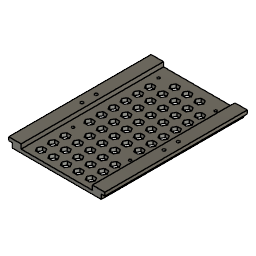
powersupply mount (Autodesk Fusion 360 design; units mm, degrees)
Autodesk Fusion 360 part; units mm, degrees
sketch "Szkic1" plane through (0, 0, 0) normal (0, 0, 1) x (1, 0, 0)
  line L0 (38.5639, 59) -> (-38.5639, 59)
  line L1 (-39, 58.5639) -> (-39, -58.5639)
  line L2 (-38.5639, -59) -> (38.5639, -59)
  line L3 (39, -58.5639) -> (39, 58.5639)
  line L4 (39, 59) -> (-39, -59) construction
  line L5 (-39, 59) -> (38.8118, -58.7152) construction
  line L6 (38.5639, 61) -> (-38.5639, 61)
  line L7 (-41, 58.5639) -> (-41, -58.5639)
  line L8 (-38.5639, -61) -> (38.5639, -61)
  line L9 (41, -58.5639) -> (41, 58.5639)
  line L10 (41, 61) -> (-41, -61) construction
  line L11 (-41, 61) -> (41, -61) construction
  line L12 (-41, 61) -> (-41, 77)
  line L13 (41, 61) -> (41, 77)
  line L14 (41, 77) -> (50, 77)
  line L15 (-41, 77) -> (-50, 77)
  line L16 (-50, 77) -> (50, 77)
  line L17 (50, 77) -> (50, -123)
  line L18 (50, -123) -> (-50, -123)
  line L19 (-50, -123) -> (-50, 77)
  circle A0 centre (-40, -60) radius 1.75
  circle A1 centre (40, -60) radius 1.75
  circle A2 centre (40, 60) radius 1.75
  circle A3 centre (-40, 60) radius 1.75
  line L20 (-67.5, -123) -> (-67.5, 77)
  line L21 (67.5, 77) -> (67.5, -123)
  line L22 (66.42, -123) -> (-67.5, 125) construction
  line L23 (-67.5, -125) -> (67.5, 125) construction
  line L24 (-67.5, 77) -> (67.5, 77)
  line L25 (-67.5, -123) -> (67.5, -123)
  line L26 (67.5, 77) -> (67.5, -123)
  line L27 (67.5, -123) -> (62.5, -123)
  line L28 (62.5, -123) -> (62.5, 77)
  line L29 (62.5, 77) -> (67.5, 77)
  line L30 (-67.5, -123) -> (-67.5, 77)
  line L31 (-67.5, 77) -> (-62.5, 77)
  line L32 (-62.5, 77) -> (-62.5, -123)
  line L33 (-62.5, -123) -> (-67.5, -123)
  dimension "d1" = 118
  dimension "d3" = 122
  dimension "d4" = 82
  dimension "d5" = 16
  dimension "d6" = 16
  dimension "d7" = 9
  dimension "d8" = 9
  dimension "d9" = 200
  dimension "d10" = 3.5
  dimension "d11" = 3.5
  dimension "d12" = 3.5
  dimension "d13" = 3.5
  dimension "d14" = 135
  dimension "d15" = 5
  dimension "d16" = 5
  constraint horizontal L0
  constraint perpendicular L0 L1
  constraint parallel L0 L2
  constraint parallel L1 L3
  constraint coincident L4 origin
  constraint coincident L5 origin
  constraint horizontal L6
  constraint perpendicular L6 L7
  constraint parallel L6 L8
  constraint parallel L7 L9
  constraint coincident L10 origin
  constraint coincident L11 origin
  constraint perpendicular L6 L12
  constraint perpendicular L6 L13
  constraint perpendicular L13 L14
  constraint perpendicular L12 L15
  constraint perpendicular L16 L17
  constraint parallel L16 L18
  constraint parallel L17 L19
  constraint coincident A0 L2.start
  constraint coincident A0 L1.end
  constraint coincident A0 L8.start
  constraint coincident A0 L7.end
  constraint coincident A1 L8.end
  constraint coincident A1 L9.start
  constraint coincident A1 L2.end
  constraint coincident A1 L5.end
  constraint coincident A1 L3.start
  constraint coincident A2 L3.end
  constraint coincident A2 L0.start
  constraint coincident A2 L6.start
  constraint coincident A2 L9.end
  constraint coincident A3 L1.start
  constraint coincident A3 L0.end
  constraint coincident A3 L7.start
  constraint coincident A3 L6.end
  constraint parallel L20 L21
  constraint coincident L22 origin
  constraint coincident L23 origin
  constraint perpendicular L21 L24
  constraint perpendicular L21 L25
  constraint coincident L25 L22.start
  constraint perpendicular L26 L27
  constraint parallel L26 L28
  constraint parallel L27 L29
  constraint perpendicular L30 L31
  constraint parallel L30 L32
  constraint parallel L31 L33
  measures "d1" distance of L5.start L4.end
  measures "d3" distance of L11.start L10.end
  measures "d4" distance of L10.end L11.end
  measures "d5" distance of L11.start L12.end
  measures "d6" distance of L10.start L13.end
  measures "d7" distance of L13.end L14.end
  measures "d8" distance of L12.end L15.end
  measures "d9" distance of L15.end L18.end
  measures "d10" diameter of A0
  measures "d11" diameter of A1
  measures "d12" diameter of A2
  measures "d13" diameter of A3
  measures "d14" distance of L22.end L23.end
  measures "d15" distance of L21.start L28.end
  measures "d16" distance of L20.start L32.end
extrude "Wyciągnięcie proste1" add sketch "Szkic1" along normal blind 4 contours L0 L1 L2 L3 A0 A1 A2 A3 | L0 L6 A2 A3 | L6 L12 L13 L16 A2 A3 L24 | L3 L9 A1 A2 | L1 L7 A0 A3 | L7 L8 L9 L12 L13 L14 L15 L16 L17 L18 L19 A0 A1 A2 A3 L24 L25 | L2 L8 A0 A1
extrude "Wyciągnięcie proste2" add 1 faces at (-13, 19.5213, 4) along direction (0, 0, 1) blind 2
extrude "Wyciągnięcie proste3" add sketch "Szkic1" along normal blind 12.5 contours L17 L24 L25 L28 | L19 L24 L25 L32 | L21 L24 L25 L26 L27 L28 L29 | L20 L24 L25 L30 L31 L32 L33
extrude "Wyciągnięcie proste4" cut sketch "Szkic1" along normal blind 7.5 contours L21 L24 L25 L26 L27 L28 L29 | L20 L24 L25 L30 L31 L32 L33
extrude "Wyciągnięcie proste5" cut 1 faces at (-13.0417, 19.4948, 0) along direction (0, 0, 1) blind 1
sketch "Szkic2" plane through (0, 0, 1) normal (0, 0, -1) x (1, 0, 0)
  line L0 (-62.5, 123) -> (-62.5, -77)
  line L1 (-62.5, -77) -> (62.5, -77)
  line L2 (62.5, -77) -> (62.5, 123)
  line L3 (62.5, 123) -> (-62.5, 123)
  circle A0 centre (-40, 60) radius 1.75
  circle A1 centre (40, -60) radius 1.75
  circle A2 centre (40, 60) radius 1.75
  circle A3 centre (-40, -60) radius 1.75
  circle A4 centre (-40, -60) radius 3
  circle A5 centre (40, -60) radius 3
  circle A6 centre (-40, 60) radius 3
  circle A7 centre (40, 60) radius 3
  dimension "d27" = 6
  dimension "d28" = 6
  dimension "d29" = 6
  dimension "d30" = 6
  constraint concentric A3 A4
  constraint concentric A1 A5
  constraint concentric A0 A6
  constraint concentric A2 A7
  measures "d27" diameter of A4
  measures "d28" diameter of A5
  measures "d29" diameter of A6
  measures "d30" diameter of A7
extrude "Wyciągnięcie proste6" cut sketch "Szkic2" against normal blind 2.4 contours A4 | A5 | A6 | A7
sketch "Szkic3" plane through (0, 0, 12.5) normal (0, 0, 1) x (-1, 0, 0)
  line L0 (50, 123) -> (50, -77)
  line L1 (50, -77) -> (67.5, -77)
  line L2 (67.5, -77) -> (67.5, 123)
  line L3 (67.5, 123) -> (50, 123)
  line L4 (50, 5) -> (60, 5)
  line L5 (50, 35) -> (50, 5)
  line L6 (60, 5) -> (62, 7)
  line L7 (62, 7) -> (62, 33)
  line L8 (62, 33) -> (60, 35)
  line L9 (60, 35) -> (50, 35)
  line L10 (-50, 35) -> (-60, 35)
  line L11 (-50, 5) -> (-50, 35)
  line L12 (-60, 35) -> (-62, 33)
  line L13 (-62, 33) -> (-62, 7)
  line L14 (-62, 7) -> (-60, 5)
  line L15 (-60, 5) -> (-50, 5)
  circle A0 centre (57.5, 30) radius 2
  circle A1 centre (57.5, 10) radius 2
  circle A2 centre (-57.5, 30) radius 2
  circle A3 centre (-57.5, 10) radius 2
  dimension "d33" = 4
  dimension "d34" = 4
  dimension "d35" = 4
  dimension "d36" = 4
  measures "d33" diameter of A0
  measures "d34" diameter of A1
  measures "d35" diameter of A2
  measures "d36" diameter of A3
extrude "Wyciągnięcie proste7" cut sketch "Szkic3" against normal blind 8 contours A0 | A1 | A2 | A3
extrude "Wyciągnięcie proste8" cut 2 faces at (58.3333, -92.6667, 12.5) (-58.3333, -92.6667, 12.5) along direction (0, 0, -1) blind 0.2
sketch "Szkic4" plane through (0, 0, 1) normal (0, 0, -1) x (1, 0, 0)
  circle A0 centre (-40, 60) radius 3
  circle A1 centre (-40, -60) radius 3
  circle A2 centre (40, 60) radius 3
  circle A3 centre (40, -60) radius 3
  line L0 (-62.5, 123) -> (-62.5, -77)
  line L1 (-62.5, -77) -> (62.5, -77)
  line L2 (62.5, -77) -> (62.5, 123)
  line L3 (62.5, 123) -> (-62.5, 123)
  line L4 (-2.8868, 30) -> (-5.7735, 25)
  line L5 (-5.7735, 25) -> (-2.8868, 20)
  line L6 (-2.8868, 20) -> (2.8868, 20)
  line L7 (2.8868, 20) -> (5.7735, 25)
  line L8 (5.7735, 25) -> (2.8868, 30)
  line L9 (2.8868, 30) -> (-2.8868, 30)
  line L10 (-37.8868, 105) -> (-32.1132, 105)
  line L11 (-40.7735, 110) -> (-37.8868, 105)
  line L12 (-37.8868, 115) -> (-40.7735, 110)
  line L13 (-32.1132, 115) -> (-37.8868, 115)
  line L14 (-29.2265, 110) -> (-32.1132, 115)
  line L15 (-32.1132, 105) -> (-29.2265, 110)
  line L16 (-20.3868, 105) -> (-14.6132, 105)
  line L17 (-23.2735, 110) -> (-20.3868, 105)
  line L18 (-20.3868, 115) -> (-23.2735, 110)
  line L19 (-14.6132, 115) -> (-20.3868, 115)
  line L20 (-11.7265, 110) -> (-14.6132, 115)
  line L21 (-14.6132, 105) -> (-11.7265, 110)
  line L22 (-2.8868, 105) -> (2.8868, 105)
  line L23 (-5.7735, 110) -> (-2.8868, 105)
  line L24 (-2.8868, 115) -> (-5.7735, 110)
  line L25 (2.8868, 115) -> (-2.8868, 115)
  line L26 (5.7735, 110) -> (2.8868, 115)
  line L27 (2.8868, 105) -> (5.7735, 110)
  line L28 (14.6132, 105) -> (20.3868, 105)
  line L29 (11.7265, 110) -> (14.6132, 105)
  line L30 (14.6132, 115) -> (11.7265, 110)
  line L31 (20.3868, 115) -> (14.6132, 115)
  line L32 (23.2735, 110) -> (20.3868, 115)
  line L33 (20.3868, 105) -> (23.2735, 110)
  line L34 (32.1132, 105) -> (37.8868, 105)
  line L35 (29.2265, 110) -> (32.1132, 105)
  line L36 (32.1132, 115) -> (29.2265, 110)
  line L37 (37.8868, 115) -> (32.1132, 115)
  line L38 (40.7735, 110) -> (37.8868, 115)
  line L39 (37.8868, 105) -> (40.7735, 110)
  line L40 (-37.8868, 88) -> (-32.1132, 88)
  line L41 (-40.7735, 93) -> (-37.8868, 88)
  line L42 (-37.8868, 98) -> (-40.7735, 93)
  line L43 (-32.1132, 98) -> (-37.8868, 98)
  line L44 (-29.2265, 93) -> (-32.1132, 98)
  line L45 (-32.1132, 88) -> (-29.2265, 93)
  line L46 (-20.3868, 88) -> (-14.6132, 88)
  line L47 (-23.2735, 93) -> (-20.3868, 88)
  line L48 (-20.3868, 98) -> (-23.2735, 93)
  line L49 (-14.6132, 98) -> (-20.3868, 98)
  line L50 (-11.7265, 93) -> (-14.6132, 98)
  line L51 (-14.6132, 88) -> (-11.7265, 93)
  line L52 (-2.8868, 88) -> (2.8868, 88)
  line L53 (-5.7735, 93) -> (-2.8868, 88)
  line L54 (-2.8868, 98) -> (-5.7735, 93)
  line L55 (2.8868, 98) -> (-2.8868, 98)
  line L56 (5.7735, 93) -> (2.8868, 98)
  line L57 (2.8868, 88) -> (5.7735, 93)
  line L58 (14.6132, 88) -> (20.3868, 88)
  line L59 (11.7265, 93) -> (14.6132, 88)
  line L60 (14.6132, 98) -> (11.7265, 93)
  line L61 (20.3868, 98) -> (14.6132, 98)
  line L62 (23.2735, 93) -> (20.3868, 98)
  line L63 (20.3868, 88) -> (23.2735, 93)
  line L64 (32.1132, 88) -> (37.8868, 88)
  line L65 (29.2265, 93) -> (32.1132, 88)
  line L66 (32.1132, 98) -> (29.2265, 93)
  line L67 (37.8868, 98) -> (32.1132, 98)
  line L68 (40.7735, 93) -> (37.8868, 98)
  line L69 (37.8868, 88) -> (40.7735, 93)
  line L70 (-37.8868, 71) -> (-32.1132, 71)
  line L71 (-40.7735, 76) -> (-37.8868, 71)
  line L72 (-37.8868, 81) -> (-40.7735, 76)
  line L73 (-32.1132, 81) -> (-37.8868, 81)
  line L74 (-29.2265, 76) -> (-32.1132, 81)
  line L75 (-32.1132, 71) -> (-29.2265, 76)
  line L76 (-20.3868, 71) -> (-14.6132, 71)
  line L77 (-23.2735, 76) -> (-20.3868, 71)
  line L78 (-20.3868, 81) -> (-23.2735, 76)
  line L79 (-14.6132, 81) -> (-20.3868, 81)
  line L80 (-11.7265, 76) -> (-14.6132, 81)
  line L81 (-14.6132, 71) -> (-11.7265, 76)
  line L82 (-2.8868, 71) -> (2.8868, 71)
  line L83 (-5.7735, 76) -> (-2.8868, 71)
  line L84 (-2.8868, 81) -> (-5.7735, 76)
  line L85 (2.8868, 81) -> (-2.8868, 81)
  line L86 (5.7735, 76) -> (2.8868, 81)
  line L87 (2.8868, 71) -> (5.7735, 76)
  line L88 (14.6132, 71) -> (20.3868, 71)
  line L89 (11.7265, 76) -> (14.6132, 71)
  line L90 (14.6132, 81) -> (11.7265, 76)
  line L91 (20.3868, 81) -> (14.6132, 81)
  line L92 (23.2735, 76) -> (20.3868, 81)
  line L93 (20.3868, 71) -> (23.2735, 76)
  line L94 (32.1132, 71) -> (37.8868, 71)
  line L95 (29.2265, 76) -> (32.1132, 71)
  line L96 (32.1132, 81) -> (29.2265, 76)
  line L97 (37.8868, 81) -> (32.1132, 81)
  line L98 (40.7735, 76) -> (37.8868, 81)
  line L99 (37.8868, 71) -> (40.7735, 76)
  line L100 (-20.3868, 54) -> (-14.6132, 54)
  line L101 (-23.2735, 59) -> (-20.3868, 54)
  line L102 (-20.3868, 64) -> (-23.2735, 59)
  line L103 (-14.6132, 64) -> (-20.3868, 64)
  line L104 (-11.7265, 59) -> (-14.6132, 64)
  line L105 (-14.6132, 54) -> (-11.7265, 59)
  line L106 (-2.8868, 54) -> (2.8868, 54)
  line L107 (-5.7735, 59) -> (-2.8868, 54)
  line L108 (-2.8868, 64) -> (-5.7735, 59)
  line L109 (2.8868, 64) -> (-2.8868, 64)
  line L110 (5.7735, 59) -> (2.8868, 64)
  line L111 (2.8868, 54) -> (5.7735, 59)
  line L112 (14.6132, 54) -> (20.3868, 54)
  line L113 (11.7265, 59) -> (14.6132, 54)
  line L114 (14.6132, 64) -> (11.7265, 59)
  line L115 (20.3868, 64) -> (14.6132, 64)
  line L116 (23.2735, 59) -> (20.3868, 64)
  line L117 (20.3868, 54) -> (23.2735, 59)
  line L118 (-37.8868, 37) -> (-32.1132, 37)
  line L119 (-40.7735, 42) -> (-37.8868, 37)
  line L120 (-37.8868, 47) -> (-40.7735, 42)
  line L121 (-32.1132, 47) -> (-37.8868, 47)
  line L122 (-29.2265, 42) -> (-32.1132, 47)
  line L123 (-32.1132, 37) -> (-29.2265, 42)
  line L124 (-20.3868, 37) -> (-14.6132, 37)
  line L125 (-23.2735, 42) -> (-20.3868, 37)
  line L126 (-20.3868, 47) -> (-23.2735, 42)
  line L127 (-14.6132, 47) -> (-20.3868, 47)
  line L128 (-11.7265, 42) -> (-14.6132, 47)
  line L129 (-14.6132, 37) -> (-11.7265, 42)
  line L130 (-2.8868, 37) -> (2.8868, 37)
  line L131 (-5.7735, 42) -> (-2.8868, 37)
  line L132 (-2.8868, 47) -> (-5.7735, 42)
  line L133 (2.8868, 47) -> (-2.8868, 47)
  line L134 (5.7735, 42) -> (2.8868, 47)
  line L135 (2.8868, 37) -> (5.7735, 42)
  line L136 (14.6132, 37) -> (20.3868, 37)
  line L137 (11.7265, 42) -> (14.6132, 37)
  line L138 (14.6132, 47) -> (11.7265, 42)
  line L139 (20.3868, 47) -> (14.6132, 47)
  line L140 (23.2735, 42) -> (20.3868, 47)
  line L141 (20.3868, 37) -> (23.2735, 42)
  line L142 (32.1132, 37) -> (37.8868, 37)
  line L143 (29.2265, 42) -> (32.1132, 37)
  line L144 (32.1132, 47) -> (29.2265, 42)
  line L145 (37.8868, 47) -> (32.1132, 47)
  line L146 (40.7735, 42) -> (37.8868, 47)
  line L147 (37.8868, 37) -> (40.7735, 42)
  line L148 (-37.8868, 20) -> (-32.1132, 20)
  line L149 (-40.7735, 25) -> (-37.8868, 20)
  line L150 (-37.8868, 30) -> (-40.7735, 25)
  line L151 (-32.1132, 30) -> (-37.8868, 30)
  line L152 (-29.2265, 25) -> (-32.1132, 30)
  line L153 (-32.1132, 20) -> (-29.2265, 25)
  line L154 (-20.3868, 20) -> (-14.6132, 20)
  line L155 (-23.2735, 25) -> (-20.3868, 20)
  line L156 (-20.3868, 30) -> (-23.2735, 25)
  line L157 (-14.6132, 30) -> (-20.3868, 30)
  line L158 (-11.7265, 25) -> (-14.6132, 30)
  line L159 (-14.6132, 20) -> (-11.7265, 25)
  line L160 (14.6132, 20) -> (20.3868, 20)
  line L161 (11.7265, 25) -> (14.6132, 20)
  line L162 (14.6132, 30) -> (11.7265, 25)
  line L163 (20.3868, 30) -> (14.6132, 30)
  line L164 (23.2735, 25) -> (20.3868, 30)
  line L165 (20.3868, 20) -> (23.2735, 25)
  line L166 (32.1132, 20) -> (37.8868, 20)
  line L167 (29.2265, 25) -> (32.1132, 20)
  line L168 (32.1132, 30) -> (29.2265, 25)
  line L169 (37.8868, 30) -> (32.1132, 30)
  line L170 (40.7735, 25) -> (37.8868, 30)
  line L171 (37.8868, 20) -> (40.7735, 25)
  line L172 (-37.8868, 3) -> (-32.1132, 3)
  line L173 (-40.7735, 8) -> (-37.8868, 3)
  line L174 (-37.8868, 13) -> (-40.7735, 8)
  line L175 (-32.1132, 13) -> (-37.8868, 13)
  line L176 (-29.2265, 8) -> (-32.1132, 13)
  line L177 (-32.1132, 3) -> (-29.2265, 8)
  line L178 (-20.3868, 3) -> (-14.6132, 3)
  line L179 (-23.2735, 8) -> (-20.3868, 3)
  line L180 (-20.3868, 13) -> (-23.2735, 8)
  line L181 (-14.6132, 13) -> (-20.3868, 13)
  line L182 (-11.7265, 8) -> (-14.6132, 13)
  line L183 (-14.6132, 3) -> (-11.7265, 8)
  line L184 (-2.8868, 3) -> (2.8868, 3)
  line L185 (-5.7735, 8) -> (-2.8868, 3)
  line L186 (-2.8868, 13) -> (-5.7735, 8)
  line L187 (2.8868, 13) -> (-2.8868, 13)
  line L188 (5.7735, 8) -> (2.8868, 13)
  line L189 (2.8868, 3) -> (5.7735, 8)
  line L190 (14.6132, 3) -> (20.3868, 3)
  line L191 (11.7265, 8) -> (14.6132, 3)
  line L192 (14.6132, 13) -> (11.7265, 8)
  line L193 (20.3868, 13) -> (14.6132, 13)
  line L194 (23.2735, 8) -> (20.3868, 13)
  line L195 (20.3868, 3) -> (23.2735, 8)
  line L196 (32.1132, 3) -> (37.8868, 3)
  line L197 (29.2265, 8) -> (32.1132, 3)
  line L198 (32.1132, 13) -> (29.2265, 8)
  line L199 (37.8868, 13) -> (32.1132, 13)
  line L200 (40.7735, 8) -> (37.8868, 13)
  line L201 (37.8868, 3) -> (40.7735, 8)
  line L202 (-37.8868, -14) -> (-32.1132, -14)
  line L203 (-40.7735, -9) -> (-37.8868, -14)
  line L204 (-37.8868, -4) -> (-40.7735, -9)
  line L205 (-32.1132, -4) -> (-37.8868, -4)
  line L206 (-29.2265, -9) -> (-32.1132, -4)
  line L207 (-32.1132, -14) -> (-29.2265, -9)
  line L208 (-20.3868, -14) -> (-14.6132, -14)
  line L209 (-23.2735, -9) -> (-20.3868, -14)
  line L210 (-20.3868, -4) -> (-23.2735, -9)
  line L211 (-14.6132, -4) -> (-20.3868, -4)
  line L212 (-11.7265, -9) -> (-14.6132, -4)
  line L213 (-14.6132, -14) -> (-11.7265, -9)
  line L214 (-2.8868, -14) -> (2.8868, -14)
  line L215 (-5.7735, -9) -> (-2.8868, -14)
  line L216 (-2.8868, -4) -> (-5.7735, -9)
  line L217 (2.8868, -4) -> (-2.8868, -4)
  line L218 (5.7735, -9) -> (2.8868, -4)
  line L219 (2.8868, -14) -> (5.7735, -9)
  line L220 (14.6132, -14) -> (20.3868, -14)
  line L221 (11.7265, -9) -> (14.6132, -14)
  line L222 (14.6132, -4) -> (11.7265, -9)
  line L223 (20.3868, -4) -> (14.6132, -4)
  line L224 (23.2735, -9) -> (20.3868, -4)
  line L225 (20.3868, -14) -> (23.2735, -9)
  line L226 (32.1132, -14) -> (37.8868, -14)
  line L227 (29.2265, -9) -> (32.1132, -14)
  line L228 (32.1132, -4) -> (29.2265, -9)
  line L229 (37.8868, -4) -> (32.1132, -4)
  line L230 (40.7735, -9) -> (37.8868, -4)
  line L231 (37.8868, -14) -> (40.7735, -9)
  line L232 (-37.8868, -31) -> (-32.1132, -31)
  line L233 (-40.7735, -26) -> (-37.8868, -31)
  line L234 (-37.8868, -21) -> (-40.7735, -26)
  line L235 (-32.1132, -21) -> (-37.8868, -21)
  line L236 (-29.2265, -26) -> (-32.1132, -21)
  line L237 (-32.1132, -31) -> (-29.2265, -26)
  line L238 (-20.3868, -31) -> (-14.6132, -31)
  line L239 (-23.2735, -26) -> (-20.3868, -31)
  line L240 (-20.3868, -21) -> (-23.2735, -26)
  line L241 (-14.6132, -21) -> (-20.3868, -21)
  line L242 (-11.7265, -26) -> (-14.6132, -21)
  line L243 (-14.6132, -31) -> (-11.7265, -26)
  line L244 (-2.8868, -31) -> (2.8868, -31)
  line L245 (-5.7735, -26) -> (-2.8868, -31)
  line L246 (-2.8868, -21) -> (-5.7735, -26)
  line L247 (2.8868, -21) -> (-2.8868, -21)
  line L248 (5.7735, -26) -> (2.8868, -21)
  line L249 (2.8868, -31) -> (5.7735, -26)
  line L250 (14.6132, -31) -> (20.3868, -31)
  line L251 (11.7265, -26) -> (14.6132, -31)
  line L252 (14.6132, -21) -> (11.7265, -26)
  line L253 (20.3868, -21) -> (14.6132, -21)
  line L254 (23.2735, -26) -> (20.3868, -21)
  line L255 (20.3868, -31) -> (23.2735, -26)
  line L256 (32.1132, -31) -> (37.8868, -31)
  line L257 (29.2265, -26) -> (32.1132, -31)
  line L258 (32.1132, -21) -> (29.2265, -26)
  line L259 (37.8868, -21) -> (32.1132, -21)
  line L260 (40.7735, -26) -> (37.8868, -21)
  line L261 (37.8868, -31) -> (40.7735, -26)
  line L262 (-37.8868, -48) -> (-32.1132, -48)
  line L263 (-40.7735, -43) -> (-37.8868, -48)
  line L264 (-37.8868, -38) -> (-40.7735, -43)
  line L265 (-32.1132, -38) -> (-37.8868, -38)
  line L266 (-29.2265, -43) -> (-32.1132, -38)
  line L267 (-32.1132, -48) -> (-29.2265, -43)
  line L268 (-20.3868, -48) -> (-14.6132, -48)
  line L269 (-23.2735, -43) -> (-20.3868, -48)
  line L270 (-20.3868, -38) -> (-23.2735, -43)
  line L271 (-14.6132, -38) -> (-20.3868, -38)
  line L272 (-11.7265, -43) -> (-14.6132, -38)
  line L273 (-14.6132, -48) -> (-11.7265, -43)
  line L274 (-2.8868, -48) -> (2.8868, -48)
  line L275 (-5.7735, -43) -> (-2.8868, -48)
  line L276 (-2.8868, -38) -> (-5.7735, -43)
  line L277 (2.8868, -38) -> (-2.8868, -38)
  line L278 (5.7735, -43) -> (2.8868, -38)
  line L279 (2.8868, -48) -> (5.7735, -43)
  line L280 (14.6132, -48) -> (20.3868, -48)
  line L281 (11.7265, -43) -> (14.6132, -48)
  line L282 (14.6132, -38) -> (11.7265, -43)
  line L283 (20.3868, -38) -> (14.6132, -38)
  line L284 (23.2735, -43) -> (20.3868, -38)
  line L285 (20.3868, -48) -> (23.2735, -43)
  line L286 (32.1132, -48) -> (37.8868, -48)
  line L287 (29.2265, -43) -> (32.1132, -48)
  line L288 (32.1132, -38) -> (29.2265, -43)
  line L289 (37.8868, -38) -> (32.1132, -38)
  line L290 (40.7735, -43) -> (37.8868, -38)
  line L291 (37.8868, -48) -> (40.7735, -43)
  line L292 (-20.3868, -65) -> (-14.6132, -65)
  line L293 (-23.2735, -60) -> (-20.3868, -65)
  line L294 (-20.3868, -55) -> (-23.2735, -60)
  line L295 (-14.6132, -55) -> (-20.3868, -55)
  line L296 (-11.7265, -60) -> (-14.6132, -55)
  line L297 (-14.6132, -65) -> (-11.7265, -60)
  line L298 (-2.8868, -65) -> (2.8868, -65)
  line L299 (-5.7735, -60) -> (-2.8868, -65)
  line L300 (-2.8868, -55) -> (-5.7735, -60)
  line L301 (2.8868, -55) -> (-2.8868, -55)
  line L302 (5.7735, -60) -> (2.8868, -55)
  line L303 (2.8868, -65) -> (5.7735, -60)
  line L304 (14.6132, -65) -> (20.3868, -65)
  line L305 (11.7265, -60) -> (14.6132, -65)
  line L306 (14.6132, -55) -> (11.7265, -60)
  line L307 (20.3868, -55) -> (14.6132, -55)
  line L308 (23.2735, -60) -> (20.3868, -55)
  line L309 (20.3868, -65) -> (23.2735, -60)
  point P0 (0, 25)
extrude "Wyciągnięcie proste9" cut sketch "Szkic4" against normal blind 100 contours L4 L5 L6 L7 L8 L9 | L10 L11 L12 L13 L14 L15 | L16 L17 L18 L19 L20 L21 | L22 L23 L24 L25 L26 L27 | L28 L29 L30 L31 L32 L33 | L34 L35 L36 L37 L38 L39 | L40 L41 L42 L43 L44 L45 | L46 L47 L48 L49 L50 L51 | L52 L53 L54 L55 L56 L57 | L58 L59 L60 L61 L62 L63 | L64 L65 L66 L67 L68 L69 | L70 L71 L72 L73 L74 L75 | L76 L77 L78 L79 L80 L81 | L82 L83 L84 L85 L86 L87 | L88 L89 L90 L91 L92 L93 | L94 L95 L96 L97 L98 L99 | L100 L101 L102 L103 L104 L105 | L106 L107 L108 L109 L110 L111 | L112 L113 L114 L115 L116 L117 | L118 L119 L120 L121 L122 L123 | L124 L125 L126 L127 L128 L129 | L130 L131 L132 L133 L134 L135 | L136 L137 L138 L139 L140 L141 | L142 L143 L144 L145 L146 L147 | L148 L149 L150 L151 L152 L153 | L154 L155 L156 L157 L158 L159 | L160 L161 L162 L163 L164 L165 | L166 L167 L168 L169 L170 L171 | L172 L173 L174 L175 L176 L177 | L178 L179 L180 L181 L182 L183 | L184 L185 L186 L187 L188 L189 | L190 L191 L192 L193 L194 L195 | L196 L197 L198 L199 L200 L201 | L202 L203 L204 L205 L206 L207 | L208 L209 L210 L211 L212 L213 | L214 L215 L216 L217 L218 L219 | L220 L221 L222 L223 L224 L225 | L226 L227 L228 L229 L230 L231 | L232 L233 L234 L235 L236 L237 | L238 L239 L240 L241 L242 L243 | L244 L245 L246 L247 L248 L249 | L250 L251 L252 L253 L254 L255 | L256 L257 L258 L259 L260 L261 | L262 L263 L264 L265 L266 L267 | L268 L269 L270 L271 L272 L273 | L274 L275 L276 L277 L278 L279 | L280 L281 L282 L283 L284 L285 | L286 L287 L288 L289 L290 L291 | L292 L293 L294 L295 L296 L297 | L298 L299 L300 L301 L302 L303 | L304 L305 L306 L307 L308 L309
